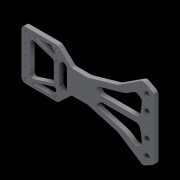
# Autodesk Inventor part: UpperArmActuatorBracket3
Saved by Autodesk Inventor 2020 (Build 240168000, 168)
## iProperties
Created: 2020-04-23
Part Number: UpperArmActuatorBracket3
Material: Generic
Document SubType Name: Sheet Metal
Designer: valer
Density: 1 g/cm^3
Flat Pattern Width: 15.7082 cm
Flat Pattern Length: 8.5309 cm
Flat Pattern Area: 134.005 cm^2
Sheet Metal Rule: Default
Sheet Metal Width: 6.184 in
Sheet Metal Length: 3.359 in
Sheet Metal Area: 20.771 in^2
Appearance: Default
Author: valer
Autodesk Inventor part; units mm, degrees
ref_plane "YZ Plane" through (0, 0, 0) normal (1, 0, 0) x (0, 1, 0)
ref_plane "XZ Plane" through (0, 0, 0) normal (0, 1, 0) x (-1, 0, 0)
ref_plane "XY Plane" through (0, 0, 0) normal (0, 0, 1) x (1, 0, 0)
sketch "Base" plane through (0, 0, 0) normal (0, 0, 1) x (1, 0, 0)
  line L0 (0, 0) -> (-64.5199, 0) construction
  line L1 (0, 0) -> (0, -36.1089)
  line L2 (-43.1523, -24.13) -> (-13.3292, -43.4974)
  line L3 (-13.3292, -43.4974) -> (0, -36.1089)
  line L4 (-43.1523, 24.13) -> (-13.3292, 43.4974)
  line L5 (-13.3292, 43.4974) -> (0, 36.1089)
  line L6 (0, 0) -> (0, 36.1089)
  line L7 (-63.823, 3.175) -> (-69.85, 9.8687)
  line L8 (-63.823, 3.175) -> (-18.103, 3.175)
  line L9 (-18.103, 3.175) -> (-15.7542, 11.3093)
  line L10 (-15.7542, 11.3093) -> (-14.4428, 23.7858)
  line L11 (-21.989, 27.9687) -> (-14.4428, 23.7858)
  line L12 (-34.0557, 20.1325) -> (-21.989, 27.9687)
  line L13 (-69.85, 9.8687) -> (-34.0557, 20.1325)
  line L14 (-43.1523, -24.13) -> (-78.74, -13.9254)
  line L15 (-43.1523, 24.13) -> (-78.74, 13.9254)
  line L16 (-106.68, 0) -> (17.78, 0) construction
  line L17 (0, -66.7984) -> (0, 66.7984) construction
  line L18 (-63.823, -3.175) -> (-69.85, -9.8687)
  line L19 (-63.823, -3.175) -> (-18.103, -3.175)
  line L20 (-69.85, -9.8687) -> (-34.0557, -20.1325)
  line L21 (-34.0557, -20.1325) -> (-21.989, -27.9687)
  line L22 (-21.989, -27.9687) -> (-14.4428, -23.7858)
  line L23 (-15.7542, -11.3093) -> (-14.4428, -23.7858)
  line L24 (-18.103, -3.175) -> (-15.7542, -11.3093)
  line L25 (-131.572, 0) -> (42.672, 0) construction
  line L26 (0, -93.5178) -> (0, 93.5178) construction
  line L27 (-76.2, -18.1203) -> (-76.2, 18.1203) construction
  line L28 (-78.74, -13.9254) -> (-78.74, 13.9254)
  line L29 (-78.74, -13.9254) -> (-85.09, -13.9254)
  line L30 (-85.09, -13.9254) -> (-85.09, 0)
  line L31 (-78.74, 13.9254) -> (-85.09, 13.9254)
  line L32 (-85.09, 13.9254) -> (-85.09, 0)
  line L33 (-78.74, -13.9254) -> (-78.74, 13.9254)
  dimension "d1" = 24.13
  dimension "d2" = 6.35
  dimension "d3" = 8.307
  dimension "d5" = 61
  dimension "d6" = 57
  dimension "d7" = 3.175
  dimension "d8" = 17.78
  dimension "d10" = 15.24
  dimension "d11" = 35.56
  dimension "d12" = 16
  dimension "d13" = 64
  dimension "d14" = 8.4667
  dimension "d15" = 45.72
  dimension "d55" = 6.35
  dimension "d56" = 6.35
  dimension "d58" = 76.2
  dimension "d66" = 2.54
  dimension "d67" = 6.35
  measures "d1" distance from line of L0 L15.start
  measures "d2" distance between parallel lines of L15 L13
  measures "d3" distance between parallel lines of L12 L4
  measures "d5" angle of L17 L5
  measures "d6" angle of L17 L4
  measures "d7" distance between parallel lines of L0 L8
  measures "d8" distance between parallel lines of L5 L11
  measures "d10" distance of L4.end L5.end
  measures "d11" distance of L15.start L4.end
  measures "d12" angle of L8 L13
  measures "d13" angle of L13 L7
  measures "d14" distance of L19.end L24.end
  measures "d15" distance of L19.start L19.end
  measures "d55" distance from line of L18.end L27
  measures "d56" distance between parallel lines of L14 L20
  measures "d58" distance between parallel lines of L17 L27
  measures "d66" distance between parallel lines of L28 L27
  measures "d67" distance of L29.start L29.end
extrude "Plate1" add sketch "Base" along normal blind 5.08
fillet "OutsideFilletsSmallFeature" radius 5.08 4 edges at (-13.3292, 43.4974, 2.54) (0, 36.1089, 2.54) (0, -36.1089, 2.54) (-13.3292, -43.4974, 2.54)
fillet "OutsideFilletsLargeFeature" radius 12.7 2 edges at (-43.1523, 24.13, 2.54) (-43.1523, -24.13, 2.54)
fillet "InsideFilletsLargeFeature" radius 5.08 10 edges at (-21.989, 27.9687, 2.54) (-14.4428, 23.7858, 2.54) (-15.7542, 11.3093, 2.54) (-63.823, 3.175, 2.54) (-18.103, 3.175, 2.54) (-18.103, -3.175, 2.54) (-15.7542, -11.3093, 2.54) (-63.823, -3.175, 2.54) (-14.4428, -23.7858, 2.54) (-21.989, -27.9687, 2.54)
fillet "InsideFilletsSmallFeature" radius 2.54 2 edges at (-69.85, 9.8687, 2.54) (-69.85, -9.8687, 2.54)
fillet "InsideFilletsLargestFeature" radius 25.4 2 edges at (-34.0557, 20.1325, 2.54) (-34.0557, -20.1325, 2.54)
sketch "ShoulderMountHoles" plane through (0, 0, 5.08) normal (0, 0, 1) x (1, 0, 0)
  line L0 (-8.4667, 31.75) -> (-8.4667, -31.75) construction
  line L1 (0, 33.1165) -> (0, -33.1165) projected
  line L2 (-2.6172, -37.5596) -> (-10.6595, -42.0175) projected
  line L3 (0, 0) -> (-84.6667, 0) construction
  circle A0 centre (-8.4667, 31.75) radius 3.175
  circle A1 centre (-8.4667, 13.97) radius 3.175
  circle A2 centre (-8.4667, -31.75) radius 3.175
  circle A3 centre (-8.4667, -13.97) radius 3.175
  point P0 (-8.4667, 0)
  dimension "d22" = 8.4667
  dimension "d24" = 63.5
  dimension "d25" = 6.35
  dimension "d26" = 17.78
  constraints: 4 centre point, 4 end point, 2 point on line, 2 symmetric about line, 1 coincident, 1 equal radius, 1 midpoint, 1 vertical, 2 other
  measures "d22" distance between parallel lines of L1 L0
  measures "d24" distance of L0.start L0.end
  measures "d25" diameter of A0
  measures "d26" distance of A3.centre L0.end
hole "ShoulderMountHolesFeature" at (-8.4667, 31.75, 5.08) at (-8.4667, 13.97, 5.08) at (-8.4667, -13.97, 5.08) at (-8.4667, -31.75, 5.08) direction (0, 0, -1) diameter 6.35 end through all
sketch "ServoMount" plane through (-154.537, -18.1203, 5.08) normal (0, 0, -1) x (-1, 0, 0)
  line L0 (-56.747, 4.1949) -> (-40.6354, -11.0451)
  line L1 (-40.6354, -11.0451) -> (2.5446, -11.0451)
  line L2 (2.5446, -11.0451) -> (2.5446, 4.1949)
  line L3 (-56.747, 32.0457) -> (-40.6354, 47.2857)
  line L4 (-40.6354, 47.2857) -> (2.5446, 47.2857)
  line L5 (2.5446, 47.2857) -> (2.5446, 32.0457)
  line L6 (-56.747, 4.1949) -> (-56.747, 32.0457)
  line L7 (2.5446, 32.0457) -> (2.5446, 4.1949)
  line L8 (2.5446, 32.0457) -> (-56.747, 32.0457) construction
  line L9 (-56.747, 4.1949) -> (2.5446, 4.1949) construction
  line L10 (31.4154, 18.1203) -> (-185.5291, 18.1203) construction
  line L11 (-69.447, 32.0457) -> (-75.797, 32.0457) construction
  line L12 (-56.747, 32.0457) -> (-69.447, 32.0457)
  line L13 (-69.447, 4.1949) -> (-69.447, 32.0457) projected
  line L14 (-56.747, 4.1949) -> (-69.447, 4.1949)
  point P0 (-154.537, 18.1203)
  point P1 (-56.747, 18.1203)
  dimension "d64" = 43.18
  dimension "d95" = 15.24
  dimension "d96" = 15.24
  dimension "d97" = 43.18
  dimension "d98" = 15.24
  dimension "d99" = 136.592
  dimension "d100" = 136.592
  dimension "d101" = 12.7
  constraints: 24 end point, 2 collinear, 2 perpendicular, 2 vertical, 1 horizontal, 1 midpoint, 1 point on line
  measures "d64" distance of L0.end L1.end
  measures "d95" vertical distance of L0.start L0.end
  measures "d96" vertical distance of L3.start L4.start
  measures "d97" distance of L4.start L5.start
  measures "d98" distance of L5.start L5.end
  measures "d99" angle of L3 L4
  measures "d100" angle of L0 L1
  measures "d101" distance of L3.start L11.start
extrude "ServoMountFeature" add sketch "ServoMount" along normal up to surface (5.08 mm away)
fillet "ServoMountOutsideFilletsFeature" radius 5.08 7 edges at (-113.9016, -29.1654, 2.54) (-113.9016, 29.1654, 2.54) (-78.74, 13.9254, 2.54) (-97.79, 13.9254, 2.54) (-97.79, -13.9254, 2.54) (-157.0816, -29.1654, 2.54) (-157.0816, 29.1654, 2.54)
sketch "ServoMountHoles" plane through (-95.6687, -12.7, 5.08) normal (0, 0, -1) x (-1, 0, 0)
  circle A0 centre (19.8683, 24.7103) radius 1.25 projected
  circle A1 centre (19.8683, 12.7103) radius 1.25 projected
  circle A2 centre (19.8683, 24.7103) radius 1.25 projected
  circle A3 centre (19.8683, 0.7103) radius 1.25 projected
  circle A4 centre (19.8683, 12.7103) radius 1.25 projected
  circle A5 centre (55.8683, -11.2897) radius 1.25 projected
  circle A6 centre (55.8683, 0.7103) radius 1.25 projected
  circle A7 centre (55.8683, 12.7103) radius 1.25 projected
  circle A8 centre (55.8683, 24.7103) radius 1.25 projected
  circle A9 centre (55.8683, 36.7103) radius 1.25 projected
  circle A10 centre (19.8683, 36.7103) radius 1.25 projected
  circle A11 centre (19.8683, -11.2897) radius 1.25 projected
  point P0 (-95.6687, 12.7)
hole "ServoMountHolesFeature" at (-115.537, 24.0103, 5.08) at (-115.537, 12.0103, 5.08) at (-115.537, 0.0103, 5.08) at (-115.537, -11.9897, 5.08) at (-115.537, -23.9897, 5.08) at (-151.537, -23.9897, 5.08) at (-151.537, -11.9897, 5.08) at (-151.537, 0.0103, 5.08) at (-151.537, 12.0103, 5.08) at (-151.537, 24.0103, 5.08) direction (0, 0, -1) diameter 2.54 end through all
sketch "ServoMountGenerative" plane through (-95.6687, -12.7, 5.08) normal (0, 0, -1) x (-1, 0, 0)
  line L0 (59.2916, 12.7) -> (-95.6687, 12.7) construction
  line L1 (50.7883, 33.5497) -> (23.0433, 24.7103)
  line L2 (23.0433, 24.7103) -> (23.0433, 12.7)
  line L3 (16.6933, 24.7103) -> (12.2191, 29.1844)
  line L4 (16.8341, 33.5497) -> (19.9838, 30.4) construction
  line L5 (19.9838, 30.4) -> (29.87, 33.5497) construction
  line L6 (29.87, 33.5497) -> (16.8341, 33.5497) construction
  line L7 (16.6933, 24.7103) -> (16.6933, 12.7)
  line L8 (16.7639, 40.4759) -> (3.5902, 28.0149) construction
  line L9 (56.3328, 41.8654) -> (20.2548, 41.8654) construction
  line L10 (7.6224, 24.8363) -> (7.6224, 12.7)
  line L11 (12.2191, 29.1844) -> (7.6224, 24.8363)
  line L12 (-95.6687, 45.8165) -> (-95.6687, -20.4165) construction
  line L13 (16.6933, 24.7103) -> (23.0433, 24.7103) construction
  line L14 (16.8341, 33.5497) -> (12.2191, 29.1844) construction
  line L15 (50.7883, 33.5497) -> (29.87, 33.5497) construction
  line L16 (50.7883, -8.1497) -> (23.0433, 0.6897)
  line L17 (23.0433, 0.6897) -> (23.0433, 12.7)
  line L18 (16.6933, 0.6897) -> (12.2191, -3.7844)
  line L19 (16.8341, -8.1497) -> (19.9838, -5) construction
  line L20 (19.9838, -5) -> (29.87, -8.1497) construction
  line L21 (29.87, -8.1497) -> (16.8341, -8.1497) construction
  line L22 (16.6933, 0.6897) -> (16.6933, 12.7)
  line L23 (7.6224, 0.5637) -> (7.6224, 12.7)
  line L24 (12.2191, -3.7844) -> (7.6224, 0.5637)
  line L25 (50.7883, 33.5497) -> (50.7883, -8.1497)
  line L26 (19.8683, 24.7103) -> (19.8683, 0.7103) construction
  circle A0 centre (19.8683, 24.7103) radius 1.27 projected
  circle A1 centre (19.8683, 0.7103) radius 1.27 projected
  circle A2 centre (55.8683, 12.7103) radius 1.27 projected
  dimension "d70" = 6.35
  dimension "d71" = 6.35
  dimension "d73" = 6.35
  dimension "d74" = 45
  dimension "d102" = 5.08
  dimension "d103" = 5.08
  constraints: 49 end point, 8 symmetric about line, 5 parallel, 3 point on line, 3 vertical, 2 collinear, 2 midpoint, 1 coincident, 1 equal length, 1 horizontal, 1 perpendicular
  measures "d70" distance between parallel lines of L5 L1
  measures "d71" distance between parallel lines of L3 L4
  measures "d73" distance between parallel lines of L7 L2
  measures "d74" angle of L0 L4
  measures "d102" distance from line of L25 A2.centre
  measures "d103" distance between parallel lines of L8 L11
extrude "ServoMountGenerativeFeature" cut sketch "ServoMountGenerative" along normal blind 25.4 contours L25 L16 L17 L2 L1 | L7 L22 L18 L24 L23 L10 L11 L3
fillet "ServoMountInsideFilletsFeature" radius 3.175 10 edges at (-118.712, 12.0103, 2.54) (-146.457, 20.8497, 2.54) (-118.712, -12.0103, 2.54) (-146.457, -20.8497, 2.54) (-112.362, -12.0103, 2.54) (-107.8879, -16.4844, 2.54) (-103.2911, -12.1363, 2.54) (-103.2911, 12.1363, 2.54) (-112.362, 12.0103, 2.54) (-107.8879, 16.4844, 2.54)
sketch "ServoMountGenerative2" plane through (-95.6687, -12.7, 5.08) normal (0, 0, -1) x (-1, 0, 0)
  line L0 (19.2813, 27.5104) -> (52.3796, 38.0554)
  line L1 (52.3796, 38.0554) -> (26.6016, 38.0554)
  line L2 (26.6016, 38.0554) -> (17.6689, 29.1228)
  line L3 (17.6689, 29.1228) -> (19.2813, 27.5104)
  line L4 (56.3328, 41.8654) -> (20.2548, 41.8654) construction
  line L5 (22.0056, -2.354) -> (54.5391, -12.6554)
  line L6 (54.5391, -12.6554) -> (26.6016, -12.6554)
  line L7 (26.6016, -12.6554) -> (19.1529, -5.2067)
  line L8 (19.1529, -5.2067) -> (22.0056, -2.354)
  line L9 (46.6494, 32.2311) -> (25.2544, 25.4147) projected
  line L10 (15.7633, 25.6402) -> (14.4026, 27.0009) projected
  circle A0 centre (19.8683, 36.7103) radius 1.27 projected
  point P0 (-95.6687, 12.7)
  dimension "d87" = 3.81
  dimension "d104" = 3.81
  dimension "d105" = 3.81
  dimension "d106" = 3.81
  constraints: 16 end point, 3 parallel, 1 perpendicular
  measures "d87" distance between parallel lines of L4 L1
  measures "d104" distance between parallel lines of L9 L0
  measures "d105" distance between parallel lines of L10 L3
  measures "d106" distance from line of A0.centre L2
extrude "ServoMountGenerative2Feature" cut sketch "ServoMountGenerative2" along normal blind 25.4 contours L3 L2 L1 L0 | L5 L6 L7 L8
fillet "ServoMountInsideFilletsSmallFeature" radius 1.27 2 edges at (-148.0484, 25.3554, 2.54) (-150.2079, -25.3554, 2.54)
fillet "ServoMountInsideFilletsLargeFeature" radius 2.54 6 edges at (-113.3377, 16.4228, 2.54) (-122.2703, 25.3554, 2.54) (-114.95, 14.8104, 2.54) (-122.2703, -25.3554, 2.54) (-117.6744, -15.054, 2.54) (-114.8216, -17.9067, 2.54)
equation "\"d7\" = 0.5 * d2"
equation "\"d32\" = Thickness"
equation "\"d80\" = Thickness"
equation "\"d71\" = d70"
equation "\"d73\" = d70"
equation "\"d16\" = Thickness"
equation "\"BendRadius\" = Thickness"
equation "\"BendReliefWidth\" = Thickness"
equation "\"BendReliefDepth\" = 0.5 * Thickness"
equation "\"CornerReliefSize\" = 4 * Thickness"
equation "\"MinimumRemnant\" = 2 * Thickness"
equation "\"TransitionRadius\" = BendRadius"
equation "\"JacobiRadiusSize\" = BendRadius"
equation "\"GapSize\" = Thickness"
equation "\"Thickness\" = 5.08"
body "Solid1"
